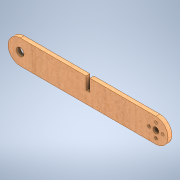
# Autodesk Inventor part: Деталь1
Saved by Autodesk Inventor 2020.1 (Build 241239000, 239)
## iProperties
Created: 2021-08-12
Part Number: Деталь1
Material: Дерево (вишня)
Document SubType Name: Modeling
Designer: Ni3na
Density: 0.63 g/cm^3
Appearance: Вишневое дерево — натуральный — со слабым глянцем
Mass: 10.276 g
Surface Area: 102.221 cm^2
Volume: 16.3111 cm^3
Author: Ni3na
Autodesk Inventor part; units mm, degrees
ref_plane "YZ Plane" through (0, 0, 0) normal (1, 0, 0) x (0, 1, 0)
ref_plane "XZ Plane" through (0, 0, 0) normal (0, 1, 0) x (-1, 0, 0)
ref_plane "XY Plane" through (0, 0, 0) normal (0, 0, 1) x (1, 0, 0)
sketch "Эскиз1" plane through (0, 0, 0) normal (0, 0, 1) x (1, 0, 0)
  circle A0 centre (0, 0) radius 12.5
  line L0 (0, -12.5) -> (140, -12.5)
  line L1 (140, -12.5) -> (140, 12.5)
  line L2 (140, 12.5) -> (0, 12.5)
  line L3 (0, 12.5) -> (0, -12.5)
  circle A1 centre (140, 0) radius 12.5
  circle A2 centre (0, 0) radius 7
  circle A3 centre (140, 0) radius 7
  circle A4 centre (0, 0) radius 4
  circle A5 centre (140, 0) radius 3
  circle A6 centre (147, 0) radius 1.5
  circle A7 centre (140, 7) radius 1.5
  circle A8 centre (140, -7) radius 1.5
  circle A9 centre (133, 0) radius 1.5
  line L4 (68, 12.5) -> (72, 12.5)
  line L5 (72, 12.5) -> (72, 0)
  line L6 (72, 0) -> (68, 0)
  line L7 (68, 0) -> (68, 12.5)
  point P0 (140, -12.5)
  point P1 (70, 12.5)
  point P2 (70, 12.5)
  point P3 (72, 12.5)
  dimension "d0" = 25
  dimension "d2" = 14
  dimension "d3" = 14
  dimension "d8" = 8
  dimension "d9" = 6
  dimension "d10" = 3
  dimension "d11" = 3
  dimension "d12" = 3
  dimension "d13" = 3
  dimension "d16" = 0
  dimension "d17" = 4
  dimension "d18" = 140
  constraints: 16 end point, 8 centre point, 5 coincident, 4 parallel, 4 point on circle, 3 midpoint, 3 point on line, 2 horizontal, 2 perpendicular, 6 other
  measures "d2" diameter of A2
  measures "d3" diameter of A3
  measures "d8" diameter of A4
  measures "d9" diameter of A5
  measures "d10" diameter of A6
  measures "d11" diameter of A7
  measures "d12" diameter of A8
  measures "d13" diameter of A9
  measures "d16" distance of point (70, 12.5) point (70, 12.5)
  measures "d17" distance of L5.end L6.end
  measures "d18" distance of point (140, 0) point (0, 0)
extrude "Выдавливание1" add sketch "Эскиз1" along normal blind 4 contours A0 L3 A2 | A0 L2 L7 L6 L5 A1 L0 | L3 A2 A0 | A2 L3 A4 | L3 A4 A2 | A1 L1 A7 A3 A9 A8 | L1 A8 A3 A6 A7 A1 | A3 A9 A7 L1 A5 A8 | L1 A5 A7 A3 A6 A8
